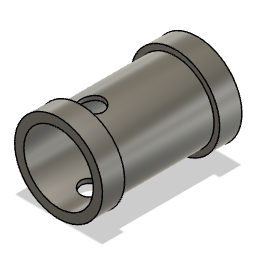
gasChargingCryoarmGuide v2 v4 (Autodesk Fusion 360 design; units mm, degrees)
Autodesk Fusion 360 part; units mm, degrees
sketch "Skizze1" plane through (0, 0, 0) normal (1, 0, 0) x (0, 0, -1)
  line L0 (-75, 0) -> (90, 0)
  line L1 (-13, 0) -> (-13, 7.9)
  line L2 (-13, 7.9) -> (-9, 7.9)
  line L3 (-9, 7.9) -> (-9, 7)
  line L4 (-9, 7) -> (8, 7)
  line L5 (8, 7) -> (8, 8)
  line L6 (8, 8) -> (12, 8)
  line L7 (12, 8) -> (12, 0)
  dimension "d1" = 7.9
  dimension "d2" = 4
  dimension "d3" = 17
  dimension "d4" = 4
  constraint horizontal L0
  constraint coincident L0 L1.start
  constraint perpendicular L0 L1
  constraint perpendicular L1 L2
  constraint perpendicular L2 L3
  constraint perpendicular L1 L4
  constraint perpendicular L4 L5
  constraint perpendicular L1 L6
  constraint coincident L0 L7.end
  constraint perpendicular L0 L7
  measures "d1" distance of L1.start L1.end
  measures "d2" distance of L1.end L2.end
  measures "d3" distance of L3.end L4.end
  measures "d4" distance of L5.end L6.end
revolve "Drehen1" add sketch "Skizze1" angle 360 about axis through (0, 0, 75) along (0, 0, -1) makes body 1
hole "Bohrung1" at (0, 0, 13) direction (0, 0, -1) diameter 12.5 end through all bodies 1
ref_plane "Arbeitsebene2" through (0, 7, 0.9561) normal (0, 1, 0) x (-1, 0, 0)
sketch "Skizze3" plane through (0, 7, 0.9561) normal (0, 1, 0) x (1, 0, 0)
  point P0 (0, -6)
hole "Bohrung2" at (0, 7, 6.9561) direction (0, -1, 0) diameter 4 depth 14 tip angle 180 bodies 1
copy_body "Körper->Berechn1" bodies 1 removing the originals makes body 2 in component "gasChargingCryoarmGuide"
component "gasChargingCryoarmGuide" placed x (1, 0, 0) y (0, 1, 0) z (0, 0, 1) at (0, 0, 0)
equation "d1 = ( 15.8 / 2 ) * 1 mm"
